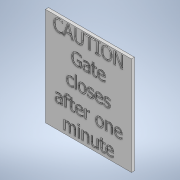
# Autodesk Inventor part: warningSignV2
Saved by Autodesk Inventor 2021.2 (Build 252289000, 289)
## iProperties
Created: 2020-11-24
Part Number: warningSignV2
Material: Generic
Document SubType Name: Modeling
Designer: robst
Density: 1 g/cm^3
Appearance: Default
Author: robst
Autodesk Inventor part; units mm, degrees
ref_plane "YZ Plane" through (0, 0, 0) normal (1, 0, 0) x (0, 1, 0)
ref_plane "XZ Plane" through (0, 0, 0) normal (0, 1, 0) x (-1, 0, 0)
ref_plane "XY Plane" through (0, 0, 0) normal (0, 0, 1) x (1, 0, 0)
sketch "Sketch4" plane through (0, 0, 0) normal (0, 0, 1) x (1, 0, 0)
  line L0 (-88.9, -101.6) -> (88.9, -101.6)
  line L1 (88.9, -101.6) -> (88.9, 101.6)
  line L2 (88.9, 101.6) -> (-88.9, 101.6)
  line L3 (-88.9, 101.6) -> (-88.9, -101.6)
  line L4 (-88.9, -101.6) -> (88.9, 101.6) construction
  line L5 (88.9, -101.6) -> (-88.9, 101.6) construction
  point P0 (0, 0)
  dimension "d12" = 203.2
  dimension "d13" = 177.8
  constraints: 12 end point, 2 midpoint, 2 parallel, 1 horizontal, 1 perpendicular
  measures "d12" distance of L2.end L0.start
  measures "d13" distance of L0.start L0.end
extrude "Extrusion2" add sketch "Sketch4" against normal blind 6.35
sketch "Sketch5" plane through (0, 0, 0) normal (0, 0, 1) x (1, 0, 0)
  line L0 (-88.9, -101.6) -> (-88.9, 101.6) construction
  line L1 (-88.9, 73.66) -> (88.9, 73.66) construction
  line L2 (88.9, 101.6) -> (88.9, -101.6) construction
  line L3 (88.9, 101.6) -> (-88.9, 101.6) construction
  spline S0 degree 2 poles (-60.6595, 73.2072) (-63.1295, 73.2072) (-67.3079, 74.8744) (-68.8311, 76.5417) knots 0 0 0 1 2 2 2
  spline S1 degree 2 poles (-68.8311, 76.5417) (-70.3543, 78.1884) (-72.0216, 83.1284) (-72.0216, 86.3394) knots 0 0 0 1 2 2 2
  spline S2 degree 2 poles (-72.0216, 86.3394) (-72.0216, 89.5299) (-70.3955, 94.2641) (-68.8517, 96.0136) knots 0 0 0 1 2 2 2
  spline S3 degree 2 poles (-68.8517, 96.0136) (-67.3285, 97.7221) (-63.1707, 99.5128) (-60.5977, 99.5128) knots 0 0 0 1 2 2 2
  spline S4 degree 2 poles (-60.5977, 99.5128) (-59.3216, 99.5128) (-57.078, 99.1423) (-56.1311, 98.8542) knots 0 0 0 1 2 2 2
  spline S5 degree 2 poles (-56.1311, 98.8542) (-55.3078, 98.5866) (-53.5993, 97.825) (-52.7554, 97.3722) knots 0 0 0 1 2 2 2
  line L4 (-52.7554, 97.3722) -> (-52.7554, 93.2966)
  line L5 (-52.7554, 93.2966) -> (-53.023, 93.2966)
  spline S6 degree 2 poles (-53.023, 93.2966) (-53.4758, 93.7083) (-54.8755, 94.861) (-55.8841, 95.4167) knots 0 0 0 1 2 2 2
  spline S7 degree 2 poles (-55.8841, 95.4167) (-56.8515, 95.9519) (-59.1363, 96.6312) (-60.6183, 96.6312) knots 0 0 0 1 2 2 2
  spline S8 degree 2 poles (-60.6183, 96.6312) (-62.2444, 96.6312) (-65.1467, 95.2932) (-66.2376, 94.017) knots 0 0 0 1 2 2 2
  spline S9 degree 2 poles (-66.2376, 94.017) (-67.3079, 92.7203) (-68.5018, 88.7888) (-68.5018, 86.3394) knots 0 0 0 1 2 2 2
  spline S10 degree 2 poles (-68.5018, 86.3394) (-68.5018, 83.7253) (-67.2462, 79.9585) (-66.1553, 78.6618) knots 0 0 0 1 2 2 2
  spline S11 degree 2 poles (-66.1553, 78.6618) (-65.0849, 77.4062) (-62.2238, 76.13) (-60.6183, 76.13) knots 0 0 0 1 2 2 2
  spline S12 degree 2 poles (-60.6183, 76.13) (-59.1569, 76.13) (-56.6663, 76.8504) (-55.6989, 77.3856) knots 0 0 0 1 2 2 2
  spline S13 degree 2 poles (-55.6989, 77.3856) (-54.7726, 77.9208) (-53.3935, 79.0323) (-53.0024, 79.4234) knots 0 0 0 1 2 2 2
  line L6 (-53.0024, 79.4234) -> (-52.7554, 79.4234)
  line L7 (-52.7554, 79.4234) -> (-52.7554, 75.389)
  spline S14 degree 2 poles (-52.7554, 75.389) (-53.5993, 74.9979) (-55.0814, 74.2775) (-56.1311, 73.9482) knots 0 0 0 1 2 2 2
  spline S15 degree 2 poles (-56.1311, 73.9482) (-57.2426, 73.5777) (-59.1363, 73.2072) (-60.6595, 73.2072) knots 0 0 0 1 2 2 2
  line L8 (-52.3438, 73.66) -> (-43.781, 99.06)
  line L9 (-43.781, 99.06) -> (-39.6232, 99.06)
  line L10 (-39.6232, 99.06) -> (-31.0605, 73.66)
  line L11 (-31.0605, 73.66) -> (-34.6214, 73.66)
  line L12 (-34.6214, 73.66) -> (-36.9267, 80.7613)
  line L13 (-36.9267, 80.7613) -> (-46.6216, 80.7613)
  line L14 (-46.6216, 80.7613) -> (-48.9269, 73.66)
  line L15 (-48.9269, 73.66) -> (-52.3438, 73.66)
  line L16 (-37.853, 83.643) -> (-41.7844, 95.602)
  line L17 (-41.7844, 95.602) -> (-45.6953, 83.643)
  line L18 (-45.6953, 83.643) -> (-37.853, 83.643)
  spline S16 degree 2 poles (-19.4514, 73.1248) (-21.695, 73.1248) (-25.0295, 74.2981) (-26.2028, 75.4713) knots 0 0 0 1 2 2 2
  spline S17 degree 2 poles (-26.2028, 75.4713) (-27.5407, 76.7887) (-28.6316, 80.4937) (-28.6316, 83.2107) knots 0 0 0 1 2 2 2
  line L19 (-28.6316, 83.2107) -> (-28.6316, 99.06)
  line L20 (-28.6316, 99.06) -> (-25.2559, 99.06)
  line L21 (-25.2559, 99.06) -> (-25.2559, 83.2107)
  spline S18 degree 2 poles (-25.2559, 83.2107) (-25.2559, 81.4406) (-24.8031, 79.0529) (-24.165, 78.0854) knots 0 0 0 1 2 2 2
  spline S19 degree 2 poles (-24.165, 78.0854) (-23.4857, 77.0563) (-21.1392, 76.0065) (-19.4514, 76.0065) knots 0 0 0 1 2 2 2
  spline S20 degree 2 poles (-19.4514, 76.0065) (-17.8665, 76.0065) (-15.3964, 77.0563) (-14.7172, 78.0854) knots 0 0 0 1 2 2 2
  spline S21 degree 2 poles (-14.7172, 78.0854) (-14.0791, 79.0529) (-13.6263, 81.42) (-13.6263, 83.1284) knots 0 0 0 1 2 2 2
  line L22 (-13.6263, 83.1284) -> (-13.6263, 99.06)
  line L23 (-13.6263, 99.06) -> (-10.2506, 99.06)
  line L24 (-10.2506, 99.06) -> (-10.2506, 83.2107)
  spline S22 degree 2 poles (-10.2506, 83.2107) (-10.2506, 80.5555) (-11.3209, 76.7681) (-12.6794, 75.4713) knots 0 0 0 1 2 2 2
  spline S23 degree 2 poles (-12.6794, 75.4713) (-13.8938, 74.2775) (-17.1049, 73.1248) (-19.4514, 73.1248) knots 0 0 0 1 2 2 2
  line L25 (0.5146, 73.66) -> (0.5146, 96.0548)
  line L26 (0.5146, 96.0548) -> (-8.007, 96.0548)
  line L27 (-8.007, 96.0548) -> (-8.007, 99.06)
  line L28 (-8.007, 99.06) -> (12.4118, 99.06)
  line L29 (12.4118, 99.06) -> (12.4118, 96.0548)
  line L30 (12.4118, 96.0548) -> (3.8903, 96.0548)
  line L31 (3.8903, 96.0548) -> (3.8903, 73.66)
  line L32 (3.8903, 73.66) -> (0.5146, 73.66)
  line L33 (23.8562, 73.66) -> (14.0173, 73.66)
  line L34 (14.0173, 73.66) -> (14.0173, 76.2535)
  line L35 (14.0173, 76.2535) -> (17.2489, 76.2535)
  line L36 (17.2489, 76.2535) -> (17.2489, 96.4665)
  line L37 (17.2489, 96.4665) -> (14.0173, 96.4665)
  line L38 (14.0173, 96.4665) -> (14.0173, 99.06)
  line L39 (14.0173, 99.06) -> (23.8562, 99.06)
  line L40 (23.8562, 99.06) -> (23.8562, 96.4665)
  line L41 (23.8562, 96.4665) -> (20.6246, 96.4665)
  line L42 (20.6246, 96.4665) -> (20.6246, 76.2535)
  line L43 (20.6246, 76.2535) -> (23.8562, 76.2535)
  line L44 (23.8562, 76.2535) -> (23.8562, 73.66)
  spline S24 degree 2 poles (46.004, 96.1577) (47.4449, 94.4699) (49.0504, 89.5299) (49.0504, 86.36) knots 0 0 0 1 2 2 2
  spline S25 degree 2 poles (49.0504, 86.36) (49.0504, 83.2725) (47.4861, 78.2707) (46.004, 76.5829) knots 0 0 0 1 2 2 2
  spline S26 degree 2 poles (46.004, 76.5829) (44.4397, 74.8127) (40.3024, 73.1248) (37.8118, 73.1248) knots 0 0 0 1 2 2 2
  spline S27 degree 2 poles (37.8118, 73.1248) (35.2389, 73.1248) (31.1222, 74.8744) (29.6196, 76.5829) knots 0 0 0 1 2 2 2
  spline S28 degree 2 poles (29.6196, 76.5829) (28.1582, 78.2707) (26.5938, 83.2313) (26.5938, 86.36) knots 0 0 0 1 2 2 2
  spline S29 degree 2 poles (26.5938, 86.36) (26.5938, 89.5504) (28.1788, 94.4081) (29.6402, 96.1577) knots 0 0 0 1 2 2 2
  spline S30 degree 2 poles (29.6402, 96.1577) (31.1222, 97.8456) (35.2595, 99.5952) (37.8118, 99.5952) knots 0 0 0 1 2 2 2
  spline S31 degree 2 poles (37.8118, 99.5952) (40.4053, 99.5952) (44.5632, 97.7838) (46.004, 96.1577) knots 0 0 0 1 2 2 2
  spline S32 degree 2 poles (45.5306, 86.36) (45.5306, 88.8712) (44.4397, 92.7615) (43.4517, 94.0376) knots 0 0 0 1 2 2 2
  spline S33 degree 2 poles (43.4517, 94.0376) (42.4431, 95.355) (39.6026, 96.6723) (37.8324, 96.6723) knots 0 0 0 1 2 2 2
  spline S34 degree 2 poles (37.8324, 96.6723) (36.0005, 96.6723) (33.2423, 95.3961) (32.1925, 94.0376) knots 0 0 0 1 2 2 2
  spline S35 degree 2 poles (32.1925, 94.0376) (31.184, 92.7409) (30.1136, 88.83) (30.1136, 86.36) knots 0 0 0 1 2 2 2
  spline S36 degree 2 poles (30.1136, 86.36) (30.1136, 81.3582) (34.3126, 76.0477) (37.8324, 76.0477) knots 0 0 0 1 2 2 2
  spline S37 degree 2 poles (37.8324, 76.0477) (41.3522, 76.0477) (45.5306, 81.3582) (45.5306, 86.36) knots 0 0 0 1 2 2 2
  line L45 (70.9306, 73.66) -> (67.1433, 73.66)
  line L46 (67.1433, 73.66) -> (55.9047, 95.5608)
  line L47 (55.9047, 95.5608) -> (55.9047, 73.66)
  line L48 (55.9047, 73.66) -> (52.7554, 73.66)
  line L49 (52.7554, 73.66) -> (52.7554, 99.06)
  line L50 (52.7554, 99.06) -> (57.5514, 99.06)
  line L51 (57.5514, 99.06) -> (67.7814, 78.95)
  line L52 (67.7814, 78.95) -> (67.7814, 99.06)
  line L53 (67.7814, 99.06) -> (70.9306, 99.06)
  line L54 (70.9306, 99.06) -> (70.9306, 73.66)
  spline S38 degree 2 poles (-22.6521, 31.3038) (-25.3485, 31.3038) (-29.8152, 32.9505) (-31.4207, 34.6177) knots 0 0 0 1 2 2 2
  spline S39 degree 2 poles (-31.4207, 34.6177) (-33.0262, 36.3056) (-34.7346, 41.2868) (-34.7346, 44.5184) knots 0 0 0 1 2 2 2
  spline S40 degree 2 poles (-34.7346, 44.5184) (-34.7346, 47.5853) (-33.0056, 52.443) (-31.4001, 54.172) knots 0 0 0 1 2 2 2
  spline S41 degree 2 poles (-31.4001, 54.172) (-29.8563, 55.8393) (-25.328, 57.6506) (-22.6315, 57.6506) knots 0 0 0 1 2 2 2
  spline S42 degree 2 poles (-22.6315, 57.6506) (-21.3348, 57.6506) (-18.9882, 57.2801) (-17.9179, 56.9508) knots 0 0 0 1 2 2 2
  spline S43 degree 2 poles (-17.9179, 56.9508) (-17.0534, 56.7038) (-14.9539, 55.7981) (-14.3158, 55.4688) knots 0 0 0 1 2 2 2
  line L55 (-14.3158, 55.4688) -> (-14.3158, 51.3933)
  line L56 (-14.3158, 51.3933) -> (-14.604, 51.3933)
  spline S44 degree 2 poles (-14.604, 51.3933) (-15.2421, 51.949) (-16.58, 52.9576) (-17.815, 53.534) knots 0 0 0 1 2 2 2
  spline S45 degree 2 poles (-17.815, 53.534) (-18.8442, 54.0485) (-21.4994, 54.7278) (-23.0226, 54.7278) knots 0 0 0 1 2 2 2
  spline S46 degree 2 poles (-23.0226, 54.7278) (-26.6865, 54.7278) (-31.2148, 49.2114) (-31.2148, 44.6213) knots 0 0 0 1 2 2 2
  spline S47 degree 2 poles (-31.2148, 44.6213) (-31.2148, 42.069) (-30.021, 38.2404) (-28.8889, 36.9231) knots 0 0 0 1 2 2 2
  spline S48 degree 2 poles (-28.8889, 36.9231) (-27.798, 35.6058) (-24.7105, 34.2267) (-22.7756, 34.2267) knots 0 0 0 1 2 2 2
  spline S49 degree 2 poles (-22.7756, 34.2267) (-21.3553, 34.2267) (-18.5148, 34.6383) (-17.5474, 35.05) knots 0 0 0 1 2 2 2
  line L57 (-17.5474, 35.05) -> (-17.5474, 41.6161)
  line L58 (-17.5474, 41.6161) -> (-23.4343, 41.6161)
  line L59 (-23.4343, 41.6161) -> (-23.4343, 44.5801)
  line L60 (-23.4343, 44.5801) -> (-14.2129, 44.5801)
  line L61 (-14.2129, 44.5801) -> (-14.2129, 33.4857)
  spline S50 degree 2 poles (-14.2129, 33.4857) (-14.851, 33.1975) (-17.0328, 32.3124) (-17.9591, 32.0448) knots 0 0 0 1 2 2 2
  spline S51 degree 2 poles (-17.9591, 32.0448) (-19.2147, 31.6743) (-21.2318, 31.3038) (-22.6521, 31.3038) knots 0 0 0 1 2 2 2
  spline S52 degree 2 poles (0.4014, 33.815) (0.0103, 33.5268) (-1.3071, 32.4976) (-1.9246, 32.1889) knots 0 0 0 1 2 2 2
  spline S53 degree 2 poles (-1.9246, 32.1889) (-2.7685, 31.7361) (-4.3534, 31.2626) (-5.7942, 31.2626) knots 0 0 0 1 2 2 2
  spline S54 degree 2 poles (-5.7942, 31.2626) (-6.9675, 31.2626) (-9.0876, 32.1477) (-9.8904, 32.9505) knots 0 0 0 1 2 2 2
  spline S55 degree 2 poles (-9.8904, 32.9505) (-10.6519, 33.7327) (-11.5782, 36.038) (-11.5782, 37.3142) knots 0 0 0 1 2 2 2
  spline S56 degree 2 poles (-11.5782, 37.3142) (-11.5782, 39.2902) (-9.9109, 42.0895) (-8.0996, 42.8923) knots 0 0 0 1 2 2 2
  spline S57 degree 2 poles (-8.0996, 42.8923) (-6.4941, 43.6333) (-2.1304, 44.1891) (0.4014, 44.3331) knots 0 0 0 1 2 2 2
  line L62 (0.4014, 44.3331) -> (0.4014, 44.9506)
  spline S58 degree 2 poles (0.4014, 44.9506) (0.4014, 46.0622) (-0.2779, 47.4412) (-0.8954, 47.8323) knots 0 0 0 1 2 2 2
  spline S59 degree 2 poles (-0.8954, 47.8323) (-1.5129, 48.2234) (-3.2831, 48.4704) (-4.2299, 48.4704) knots 0 0 0 1 2 2 2
  spline S60 degree 2 poles (-4.2299, 48.4704) (-5.3414, 48.4704) (-8.3466, 47.8117) (-9.8492, 47.1737) knots 0 0 0 1 2 2 2
  line L63 (-9.8492, 47.1737) -> (-10.0344, 47.1737)
  line L64 (-10.0344, 47.1737) -> (-10.0344, 50.4464)
  spline S61 degree 2 poles (-10.0344, 50.4464) (-9.1494, 50.6934) (-5.8354, 51.3109) (-4.2093, 51.3109) knots 0 0 0 1 2 2 2
  spline S62 degree 2 poles (-4.2093, 51.3109) (-2.2333, 51.3109) (0.4631, 50.6934) (1.5335, 49.8907) knots 0 0 0 1 2 2 2
  spline S63 degree 2 poles (1.5335, 49.8907) (2.5832, 49.1085) (3.6124, 46.6179) (3.6124, 44.8271) knots 0 0 0 1 2 2 2
  line L65 (3.6124, 44.8271) -> (3.6124, 31.7978)
  line L66 (3.6124, 31.7978) -> (0.4014, 31.7978)
  line L67 (0.4014, 31.7978) -> (0.4014, 33.815)
  line L68 (0.4014, 36.4908) -> (0.4014, 41.7808)
  spline S64 degree 2 poles (0.4014, 41.7808) (-0.7513, 41.6779) (-4.2299, 41.328) (-5.3208, 40.9986) knots 0 0 0 1 2 2 2
  spline S65 degree 2 poles (-5.3208, 40.9986) (-6.597, 40.6075) (-8.2643, 38.9814) (-8.2643, 37.5406) knots 0 0 0 1 2 2 2
  spline S66 degree 2 poles (-8.2643, 37.5406) (-8.2643, 35.8939) (-6.4118, 34.2267) (-4.6416, 34.2267) knots 0 0 0 1 2 2 2
  spline S67 degree 2 poles (-4.6416, 34.2267) (-3.139, 34.2267) (-0.669, 35.5234) (0.4014, 36.4908) knots 0 0 0 1 2 2 2
  spline S68 degree 2 poles (13.8835, 31.4273) (11.2694, 31.4273) (8.326, 34.4119) (8.326, 37.6435) knots 0 0 0 1 2 2 2
  line L69 (8.326, 37.6435) -> (8.326, 48.2028)
  line L70 (8.326, 48.2028) -> (6.1647, 48.2028)
  line L71 (6.1647, 48.2028) -> (6.1647, 50.8581)
  line L72 (6.1647, 50.8581) -> (8.326, 50.8581)
  line L73 (8.326, 50.8581) -> (8.326, 56.3333)
  line L74 (8.326, 56.3333) -> (11.537, 56.3333)
  line L75 (11.537, 56.3333) -> (11.537, 50.8581)
  line L76 (11.537, 50.8581) -> (17.4445, 50.8581)
  line L77 (17.4445, 50.8581) -> (17.4445, 48.2028)
  line L78 (17.4445, 48.2028) -> (11.537, 48.2028)
  line L79 (11.537, 48.2028) -> (11.537, 39.1255)
  spline S69 degree 2 poles (11.537, 39.1255) (11.537, 37.6847) (11.64, 36.0998) (11.9899, 35.4205) knots 0 0 0 1 2 2 2
  spline S70 degree 2 poles (11.9899, 35.4205) (12.278, 34.8236) (13.5748, 34.2267) (14.6863, 34.2267) knots 0 0 0 1 2 2 2
  spline S71 degree 2 poles (14.6863, 34.2267) (15.4685, 34.2267) (16.9299, 34.7001) (17.2592, 34.8442) knots 0 0 0 1 2 2 2
  line L80 (17.2592, 34.8442) -> (17.4445, 34.8442)
  line L81 (17.4445, 34.8442) -> (17.4445, 31.9625)
  spline S72 degree 2 poles (17.4445, 31.9625) (16.5388, 31.7155) (14.6863, 31.4273) (13.8835, 31.4273) knots 0 0 0 1 2 2 2
  spline S73 degree 2 poles (28.0861, 31.3656) (23.5166, 31.3656) (18.4942, 36.4908) (18.4942, 41.225) knots 0 0 0 1 2 2 2
  spline S74 degree 2 poles (18.4942, 41.225) (18.4942, 45.8769) (23.3725, 51.3933) (27.304, 51.3933) knots 0 0 0 1 2 2 2
  spline S75 degree 2 poles (27.304, 51.3933) (29.0741, 51.3933) (31.8117, 50.3641) (32.8203, 49.2732) knots 0 0 0 1 2 2 2
  spline S76 degree 2 poles (32.8203, 49.2732) (33.8495, 48.1823) (34.9404, 45.033) (34.9404, 42.7482) knots 0 0 0 1 2 2 2
  line L82 (34.9404, 42.7482) -> (34.9404, 40.9986)
  line L83 (34.9404, 40.9986) -> (21.7464, 40.9986)
  spline S77 degree 2 poles (21.7464, 40.9986) (21.7464, 37.6847) (25.081, 34.1649) (28.045, 34.1649) knots 0 0 0 1 2 2 2
  spline S78 degree 2 poles (28.045, 34.1649) (29.0947, 34.1649) (31.1325, 34.6383) (31.9558, 35.0088) knots 0 0 0 1 2 2 2
  spline S79 degree 2 poles (31.9558, 35.0088) (32.8203, 35.4205) (34.0142, 36.1409) (34.4053, 36.4703) knots 0 0 0 1 2 2 2
  line L84 (34.4053, 36.4703) -> (34.5905, 36.4703)
  line L85 (34.5905, 36.4703) -> (34.5905, 32.9711)
  spline S80 degree 2 poles (34.5905, 32.9711) (34.0348, 32.7446) (32.3469, 32.086) (31.6882, 31.9007) knots 0 0 0 1 2 2 2
  spline S81 degree 2 poles (31.6882, 31.9007) (30.762, 31.6331) (29.2388, 31.3656) (28.0861, 31.3656) knots 0 0 0 1 2 2 2
  spline S82 degree 2 poles (31.8117, 43.4481) (31.7706, 44.7448) (31.2354, 46.6385) (30.7208, 47.2766) knots 0 0 0 1 2 2 2
  spline S83 degree 2 poles (30.7208, 47.2766) (30.1651, 47.997) (28.4155, 48.7586) (27.1187, 48.7586) knots 0 0 0 1 2 2 2
  spline S84 degree 2 poles (27.1187, 48.7586) (25.8425, 48.7586) (24.0518, 47.997) (23.3108, 47.256) knots 0 0 0 1 2 2 2
  spline S85 degree 2 poles (23.3108, 47.256) (22.5904, 46.4944) (21.8494, 44.6625) (21.7464, 43.4481) knots 0 0 0 1 2 2 2
  line L86 (21.7464, 43.4481) -> (31.8117, 43.4481)
  spline S86 degree 2 poles (-36.4019, -11.1759) (-38.3779, -11.1759) (-41.6506, -9.9615) (-42.8239, -8.7265) knots 0 0 0 1 2 2 2
  spline S87 degree 2 poles (-42.8239, -8.7265) (-43.9972, -7.512) (-45.2939, -3.7658) (-45.2939, -1.2547) knots 0 0 0 1 2 2 2
  spline S88 degree 2 poles (-45.2939, -1.2547) (-45.2939, 1.2565) (-43.956, 4.9204) (-42.8239, 6.1554) knots 0 0 0 1 2 2 2
  spline S89 degree 2 poles (-42.8239, 6.1554) (-41.6918, 7.411) (-38.3367, 8.7489) (-36.4019, 8.7489) knots 0 0 0 1 2 2 2
  spline S90 degree 2 poles (-36.4019, 8.7489) (-34.8375, 8.7489) (-31.9147, 7.8638) (-30.7826, 7.2875) knots 0 0 0 1 2 2 2
  line L87 (-30.7826, 7.2875) -> (-30.7826, 3.6854)
  line L88 (-30.7826, 3.6854) -> (-30.9678, 3.6854)
  spline S91 degree 2 poles (-30.9678, 3.6854) (-31.3177, 3.9735) (-32.3881, 4.7146) (-33.1497, 5.1056) knots 0 0 0 1 2 2 2
  spline S92 degree 2 poles (-33.1497, 5.1056) (-33.8289, 5.435) (-35.6403, 5.9496) (-36.4636, 5.9496) knots 0 0 0 1 2 2 2
  spline S93 degree 2 poles (-36.4636, 5.9496) (-38.9542, 5.9496) (-41.98, 2.1828) (-41.98, -1.2547) knots 0 0 0 1 2 2 2
  spline S94 degree 2 poles (-41.98, -1.2547) (-41.98, -4.6098) (-39.0571, -8.3765) (-36.4636, -8.3765) knots 0 0 0 1 2 2 2
  spline S95 degree 2 poles (-36.4636, -8.3765) (-34.8993, -8.3765) (-32.0587, -7.0798) (-30.9678, -6.0712) knots 0 0 0 1 2 2 2
  line L89 (-30.9678, -6.0712) -> (-30.7826, -6.0712)
  line L90 (-30.7826, -6.0712) -> (-30.7826, -9.6733)
  spline S96 degree 2 poles (-30.7826, -9.6733) (-31.256, -9.8997) (-32.6968, -10.5378) (-33.2732, -10.6819) knots 0 0 0 1 2 2 2
  spline S97 degree 2 poles (-33.2732, -10.6819) (-34.0965, -10.9289) (-35.3933, -11.1759) (-36.4019, -11.1759) knots 0 0 0 1 2 2 2
  line L91 (-24.587, -10.7436) -> (-27.798, -10.7436)
  line L92 (-27.798, -10.7436) -> (-27.798, 15.7885)
  line L93 (-27.798, 15.7885) -> (-24.587, 15.7885)
  line L94 (-24.587, 15.7885) -> (-24.587, -10.7436)
  spline S98 degree 2 poles (-4.2093, -1.2135) (-4.2093, -6.03) (-8.8406, -11.2788) (-12.7103, -11.2788) knots 0 0 0 1 2 2 2
  spline S99 degree 2 poles (-12.7103, -11.2788) (-16.6829, -11.2788) (-21.2318, -5.8654) (-21.2318, -1.2135) knots 0 0 0 1 2 2 2
  spline S100 degree 2 poles (-21.2318, -1.2135) (-21.2318, 3.5619) (-16.5388, 8.8518) (-12.7103, 8.8518) knots 0 0 0 1 2 2 2
  spline S101 degree 2 poles (-12.7103, 8.8518) (-8.8406, 8.8518) (-4.2093, 3.5825) (-4.2093, -1.2135) knots 0 0 0 1 2 2 2
  spline S102 degree 2 poles (-7.5233, -1.2135) (-7.5233, 2.4915) (-10.2197, 6.0936) (-12.7103, 6.0936) knots 0 0 0 1 2 2 2
  spline S103 degree 2 poles (-12.7103, 6.0936) (-15.2009, 6.0936) (-17.9179, 2.4915) (-17.9179, -1.2135) knots 0 0 0 1 2 2 2
  spline S104 degree 2 poles (-17.9179, -1.2135) (-17.9179, -4.8156) (-15.2009, -8.5206) (-12.7103, -8.5206) knots 0 0 0 1 2 2 2
  spline S105 degree 2 poles (-12.7103, -8.5206) (-10.2403, -8.5206) (-7.5233, -4.8773) (-7.5233, -1.2135) knots 0 0 0 1 2 2 2
  spline S106 degree 2 poles (4.2299, -11.1965) (2.3156, -11.1965) (-0.9983, -10.1673) (-2.0892, -9.591) knots 0 0 0 1 2 2 2
  line L95 (-2.0892, -9.591) -> (-2.0892, -5.9889)
  line L96 (-2.0892, -5.9889) -> (-1.9246, -5.9889)
  spline S107 degree 2 poles (-1.9246, -5.9889) (-1.5129, -6.3182) (-0.4014, -7.1004) (0.5249, -7.5326) knots 0 0 0 1 2 2 2
  spline S108 degree 2 poles (0.5249, -7.5326) (1.3276, -7.9237) (3.3036, -8.5) (4.3534, -8.5) knots 0 0 0 1 2 2 2
  spline S109 degree 2 poles (4.3534, -8.5) (5.115, -8.5) (6.8646, -8.1501) (7.2763, -7.8619) knots 0 0 0 1 2 2 2
  spline S110 degree 2 poles (7.2763, -7.8619) (7.8732, -7.4709) (8.4083, -6.5858) (8.4083, -5.6801) knots 0 0 0 1 2 2 2
  spline S111 degree 2 poles (8.4083, -5.6801) (8.4083, -4.548) (7.1733, -3.3748) (5.5884, -2.9837) knots 0 0 0 1 2 2 2
  spline S112 degree 2 poles (5.5884, -2.9837) (4.9709, -2.8396) (2.9949, -2.4279) (2.151, -2.2015) knots 0 0 0 1 2 2 2
  spline S113 degree 2 poles (2.151, -2.2015) (-0.0309, -1.5634) (-2.0069, 1.0713) (-2.0069, 2.9444) knots 0 0 0 1 2 2 2
  spline S114 degree 2 poles (-2.0069, 2.9444) (-2.0069, 5.5379) (1.8834, 8.7695) (5.0944, 8.7695) knots 0 0 0 1 2 2 2
  spline S115 degree 2 poles (5.0944, 8.7695) (6.6793, 8.7695) (9.8904, 7.9873) (10.9813, 7.3904) knots 0 0 0 1 2 2 2
  line L97 (10.9813, 7.3904) -> (10.9813, 3.953)
  line L98 (10.9813, 3.953) -> (10.8166, 3.953)
  spline S116 degree 2 poles (10.8166, 3.953) (9.5816, 4.941) (6.5764, 6.0731) (5.0327, 6.0731) knots 0 0 0 1 2 2 2
  spline S117 degree 2 poles (5.0327, 6.0731) (3.4477, 6.0731) (1.2659, 4.7351) (1.2659, 3.3972) knots 0 0 0 1 2 2 2
  spline S118 degree 2 poles (1.2659, 3.3972) (1.2659, 2.1828) (2.5626, 1.0095) (4.0035, 0.639) knots 0 0 0 1 2 2 2
  spline S119 degree 2 poles (4.0035, 0.639) (4.7033, 0.4538) (6.4735, 0.0833) (7.4409, -0.1431) knots 0 0 0 1 2 2 2
  spline S120 degree 2 poles (7.4409, -0.1431) (9.5404, -0.6783) (11.6811, -3.1278) (11.6811, -5.2478) knots 0 0 0 1 2 2 2
  spline S121 degree 2 poles (11.6811, -5.2478) (11.6811, -6.4829) (10.7137, -8.6647) (9.7669, -9.4675) knots 0 0 0 1 2 2 2
  spline S122 degree 2 poles (9.7669, -9.4675) (8.7583, -10.3114) (6.1853, -11.1965) (4.2299, -11.1965) knots 0 0 0 1 2 2 2
  spline S123 degree 2 poles (22.9403, -11.1759) (18.3707, -11.1759) (13.3484, -6.0506) (13.3484, -1.3164) knots 0 0 0 1 2 2 2
  spline S124 degree 2 poles (13.3484, -1.3164) (13.3484, 3.3355) (18.2267, 8.8518) (22.1581, 8.8518) knots 0 0 0 1 2 2 2
  spline S125 degree 2 poles (22.1581, 8.8518) (23.9283, 8.8518) (26.6659, 7.8227) (27.6745, 6.7317) knots 0 0 0 1 2 2 2
  spline S126 degree 2 poles (27.6745, 6.7317) (28.7036, 5.6408) (29.7946, 2.4915) (29.7946, 0.2068) knots 0 0 0 1 2 2 2
  line L99 (29.7946, 0.2068) -> (29.7946, -1.5428)
  line L100 (29.7946, -1.5428) -> (16.6006, -1.5428)
  spline S127 degree 2 poles (16.6006, -1.5428) (16.6006, -4.8568) (19.9351, -8.3765) (22.8991, -8.3765) knots 0 0 0 1 2 2 2
  spline S128 degree 2 poles (22.8991, -8.3765) (23.9489, -8.3765) (25.9866, -7.9031) (26.81, -7.5326) knots 0 0 0 1 2 2 2
  spline S129 degree 2 poles (26.81, -7.5326) (27.6745, -7.1209) (28.8683, -6.4005) (29.2594, -6.0712) knots 0 0 0 1 2 2 2
  line L101 (29.2594, -6.0712) -> (29.4447, -6.0712)
  line L102 (29.4447, -6.0712) -> (29.4447, -9.5704)
  spline S130 degree 2 poles (29.4447, -9.5704) (28.8889, -9.7968) (27.2011, -10.4555) (26.5424, -10.6407) knots 0 0 0 1 2 2 2
  spline S131 degree 2 poles (26.5424, -10.6407) (25.6161, -10.9083) (24.093, -11.1759) (22.9403, -11.1759) knots 0 0 0 1 2 2 2
  spline S132 degree 2 poles (26.6659, 0.9066) (26.6247, 2.2034) (26.0895, 4.097) (25.575, 4.7351) knots 0 0 0 1 2 2 2
  spline S133 degree 2 poles (25.575, 4.7351) (25.0192, 5.4556) (23.2696, 6.2171) (21.9729, 6.2171) knots 0 0 0 1 2 2 2
  spline S134 degree 2 poles (21.9729, 6.2171) (20.6967, 6.2171) (18.9059, 5.4556) (18.1649, 4.7146) knots 0 0 0 1 2 2 2
  spline S135 degree 2 poles (18.1649, 4.7146) (17.4445, 3.953) (16.7035, 2.121) (16.6006, 0.9066) knots 0 0 0 1 2 2 2
  line L103 (16.6006, 0.9066) -> (26.6659, 0.9066)
  spline S136 degree 2 poles (38.1926, -11.1965) (36.2784, -11.1965) (32.9644, -10.1673) (31.8735, -9.591) knots 0 0 0 1 2 2 2
  line L104 (31.8735, -9.591) -> (31.8735, -5.9889)
  line L105 (31.8735, -5.9889) -> (32.0382, -5.9889)
  spline S137 degree 2 poles (32.0382, -5.9889) (32.4498, -6.3182) (33.5613, -7.1004) (34.4876, -7.5326) knots 0 0 0 1 2 2 2
  spline S138 degree 2 poles (34.4876, -7.5326) (35.2904, -7.9237) (37.2664, -8.5) (38.3161, -8.5) knots 0 0 0 1 2 2 2
  spline S139 degree 2 poles (38.3161, -8.5) (39.0777, -8.5) (40.8273, -8.1501) (41.239, -7.8619) knots 0 0 0 1 2 2 2
  spline S140 degree 2 poles (41.239, -7.8619) (41.8359, -7.4709) (42.3711, -6.5858) (42.3711, -5.6801) knots 0 0 0 1 2 2 2
  spline S141 degree 2 poles (42.3711, -5.6801) (42.3711, -4.548) (41.1361, -3.3748) (39.5511, -2.9837) knots 0 0 0 1 2 2 2
  spline S142 degree 2 poles (39.5511, -2.9837) (38.9336, -2.8396) (36.9576, -2.4279) (36.1137, -2.2015) knots 0 0 0 1 2 2 2
  spline S143 degree 2 poles (36.1137, -2.2015) (33.9318, -1.5634) (31.9558, 1.0713) (31.9558, 2.9444) knots 0 0 0 1 2 2 2
  spline S144 degree 2 poles (31.9558, 2.9444) (31.9558, 5.5379) (35.8461, 8.7695) (39.0571, 8.7695) knots 0 0 0 1 2 2 2
  spline S145 degree 2 poles (39.0571, 8.7695) (40.6421, 8.7695) (43.8531, 7.9873) (44.944, 7.3904) knots 0 0 0 1 2 2 2
  line L106 (44.944, 7.3904) -> (44.944, 3.953)
  line L107 (44.944, 3.953) -> (44.7793, 3.953)
  spline S146 degree 2 poles (44.7793, 3.953) (43.5443, 4.941) (40.5391, 6.0731) (38.9954, 6.0731) knots 0 0 0 1 2 2 2
  spline S147 degree 2 poles (38.9954, 6.0731) (37.4105, 6.0731) (35.2286, 4.7351) (35.2286, 3.3972) knots 0 0 0 1 2 2 2
  spline S148 degree 2 poles (35.2286, 3.3972) (35.2286, 2.1828) (36.5254, 1.0095) (37.9662, 0.639) knots 0 0 0 1 2 2 2
  spline S149 degree 2 poles (37.9662, 0.639) (38.666, 0.4538) (40.4362, 0.0833) (41.4036, -0.1431) knots 0 0 0 1 2 2 2
  spline S150 degree 2 poles (41.4036, -0.1431) (43.5032, -0.6783) (45.6438, -3.1278) (45.6438, -5.2478) knots 0 0 0 1 2 2 2
  spline S151 degree 2 poles (45.6438, -5.2478) (45.6438, -6.4829) (44.6764, -8.6647) (43.7296, -9.4675) knots 0 0 0 1 2 2 2
  spline S152 degree 2 poles (43.7296, -9.4675) (42.721, -10.3114) (40.1481, -11.1965) (38.1926, -11.1965) knots 0 0 0 1 2 2 2
  spline S153 degree 2 poles (-56.975, -51.4326) (-57.3661, -51.7207) (-58.6835, -52.7499) (-59.301, -53.0587) knots 0 0 0 1 2 2 2
  spline S154 degree 2 poles (-59.301, -53.0587) (-60.1449, -53.5115) (-61.7298, -53.9849) (-63.1707, -53.9849) knots 0 0 0 1 2 2 2
  spline S155 degree 2 poles (-63.1707, -53.9849) (-64.3439, -53.9849) (-66.464, -53.0998) (-67.2668, -52.2971) knots 0 0 0 1 2 2 2
  spline S156 degree 2 poles (-67.2668, -52.2971) (-68.0284, -51.5149) (-68.9546, -49.2096) (-68.9546, -47.9334) knots 0 0 0 1 2 2 2
  spline S157 degree 2 poles (-68.9546, -47.9334) (-68.9546, -45.9574) (-67.2874, -43.158) (-65.476, -42.3553) knots 0 0 0 1 2 2 2
  spline S158 degree 2 poles (-65.476, -42.3553) (-63.8705, -41.6143) (-59.5068, -41.0585) (-56.975, -40.9144) knots 0 0 0 1 2 2 2
  line L108 (-56.975, -40.9144) -> (-56.975, -40.2969)
  spline S159 degree 2 poles (-56.975, -40.2969) (-56.975, -39.1854) (-57.6543, -37.8063) (-58.2718, -37.4152) knots 0 0 0 1 2 2 2
  spline S160 degree 2 poles (-58.2718, -37.4152) (-58.8893, -37.0241) (-60.6595, -36.7771) (-61.6063, -36.7771) knots 0 0 0 1 2 2 2
  spline S161 degree 2 poles (-61.6063, -36.7771) (-62.7178, -36.7771) (-65.723, -37.4358) (-67.2256, -38.0739) knots 0 0 0 1 2 2 2
  line L109 (-67.2256, -38.0739) -> (-67.4109, -38.0739)
  line L110 (-67.4109, -38.0739) -> (-67.4109, -34.8011)
  spline S162 degree 2 poles (-67.4109, -34.8011) (-66.5258, -34.5541) (-63.2118, -33.9366) (-61.5857, -33.9366) knots 0 0 0 1 2 2 2
  spline S163 degree 2 poles (-61.5857, -33.9366) (-59.6097, -33.9366) (-56.9133, -34.5541) (-55.8429, -35.3569) knots 0 0 0 1 2 2 2
  spline S164 degree 2 poles (-55.8429, -35.3569) (-54.7932, -36.1391) (-53.764, -38.6296) (-53.764, -40.4204) knots 0 0 0 1 2 2 2
  line L111 (-53.764, -40.4204) -> (-53.764, -53.4497)
  line L112 (-53.764, -53.4497) -> (-56.975, -53.4497)
  line L113 (-56.975, -53.4497) -> (-56.975, -51.4326)
  line L114 (-56.975, -48.7567) -> (-56.975, -43.4668)
  spline S165 degree 2 poles (-56.975, -43.4668) (-58.1277, -43.5697) (-61.6063, -43.9196) (-62.6972, -44.2489) knots 0 0 0 1 2 2 2
  spline S166 degree 2 poles (-62.6972, -44.2489) (-63.9734, -44.64) (-65.6407, -46.2661) (-65.6407, -47.707) knots 0 0 0 1 2 2 2
  spline S167 degree 2 poles (-65.6407, -47.707) (-65.6407, -49.3536) (-63.7882, -51.0209) (-62.018, -51.0209) knots 0 0 0 1 2 2 2
  spline S168 degree 2 poles (-62.018, -51.0209) (-60.5154, -51.0209) (-58.0454, -49.7241) (-56.975, -48.7567) knots 0 0 0 1 2 2 2
  line L115 (-39.2321, -30.0052) -> (-39.3968, -30.0052)
  spline S169 degree 2 poles (-39.3968, -30.0052) (-39.829, -29.8405) (-41.4345, -29.5523) (-42.0726, -29.5523) knots 0 0 0 1 2 2 2
  spline S170 degree 2 poles (-42.0726, -29.5523) (-44.0898, -29.5523) (-45.8188, -31.3637) (-45.8188, -33.7514) knots 0 0 0 1 2 2 2
  line L116 (-45.8188, -33.7514) -> (-45.8188, -34.3895)
  line L117 (-45.8188, -34.3895) -> (-40.5083, -34.3895)
  line L118 (-40.5083, -34.3895) -> (-40.5083, -37.0447)
  line L119 (-40.5083, -37.0447) -> (-45.7159, -37.0447)
  line L120 (-45.7159, -37.0447) -> (-45.7159, -53.4497)
  line L121 (-45.7159, -53.4497) -> (-48.9269, -53.4497)
  line L122 (-48.9269, -53.4497) -> (-48.9269, -37.0447)
  line L123 (-48.9269, -37.0447) -> (-51.0882, -37.0447)
  line L124 (-51.0882, -37.0447) -> (-51.0882, -34.3895)
  line L125 (-51.0882, -34.3895) -> (-48.9269, -34.3895)
  line L126 (-48.9269, -34.3895) -> (-48.9269, -33.7514)
  spline S171 degree 2 poles (-48.9269, -33.7514) (-48.9269, -30.3345) (-45.613, -26.753) (-42.5254, -26.753) knots 0 0 0 1 2 2 2
  spline S172 degree 2 poles (-42.5254, -26.753) (-41.6404, -26.753) (-39.9319, -26.9382) (-39.2321, -27.0617) knots 0 0 0 1 2 2 2
  line L127 (-39.2321, -27.0617) -> (-39.2321, -30.0052)
  spline S173 degree 2 poles (-31.6368, -53.8202) (-34.2509, -53.8202) (-37.1943, -50.8356) (-37.1943, -47.604) knots 0 0 0 1 2 2 2
  line L128 (-37.1943, -47.604) -> (-37.1943, -37.0447)
  line L129 (-37.1943, -37.0447) -> (-39.3556, -37.0447)
  line L130 (-39.3556, -37.0447) -> (-39.3556, -34.3895)
  line L131 (-39.3556, -34.3895) -> (-37.1943, -34.3895)
  line L132 (-37.1943, -34.3895) -> (-37.1943, -28.9143)
  line L133 (-37.1943, -28.9143) -> (-33.9833, -28.9143)
  line L134 (-33.9833, -28.9143) -> (-33.9833, -34.3895)
  line L135 (-33.9833, -34.3895) -> (-28.0758, -34.3895)
  line L136 (-28.0758, -34.3895) -> (-28.0758, -37.0447)
  line L137 (-28.0758, -37.0447) -> (-33.9833, -37.0447)
  line L138 (-33.9833, -37.0447) -> (-33.9833, -46.122)
  spline S174 degree 2 poles (-33.9833, -46.122) (-33.9833, -47.5629) (-33.8804, -49.1478) (-33.5305, -49.8271) knots 0 0 0 1 2 2 2
  spline S175 degree 2 poles (-33.5305, -49.8271) (-33.2423, -50.424) (-31.9455, -51.0209) (-30.834, -51.0209) knots 0 0 0 1 2 2 2
  spline S176 degree 2 poles (-30.834, -51.0209) (-30.0519, -51.0209) (-28.5904, -50.5475) (-28.2611, -50.4034) knots 0 0 0 1 2 2 2
  line L139 (-28.2611, -50.4034) -> (-28.0758, -50.4034)
  line L140 (-28.0758, -50.4034) -> (-28.0758, -53.2851)
  spline S177 degree 2 poles (-28.0758, -53.2851) (-28.9815, -53.5321) (-30.834, -53.8202) (-31.6368, -53.8202) knots 0 0 0 1 2 2 2
  spline S178 degree 2 poles (-17.4342, -53.882) (-22.0037, -53.882) (-27.0261, -48.7567) (-27.0261, -44.0225) knots 0 0 0 1 2 2 2
  spline S179 degree 2 poles (-27.0261, -44.0225) (-27.0261, -39.3707) (-22.1478, -33.8543) (-18.2164, -33.8543) knots 0 0 0 1 2 2 2
  spline S180 degree 2 poles (-18.2164, -33.8543) (-16.4462, -33.8543) (-13.7086, -34.8835) (-12.7, -35.9744) knots 0 0 0 1 2 2 2
  spline S181 degree 2 poles (-12.7, -35.9744) (-11.6708, -37.0653) (-10.5799, -40.2146) (-10.5799, -42.4993) knots 0 0 0 1 2 2 2
  line L141 (-10.5799, -42.4993) -> (-10.5799, -44.2489)
  line L142 (-10.5799, -44.2489) -> (-23.7739, -44.2489)
  spline S182 degree 2 poles (-23.7739, -44.2489) (-23.7739, -47.5629) (-20.4394, -51.0826) (-17.4754, -51.0826) knots 0 0 0 1 2 2 2
  spline S183 degree 2 poles (-17.4754, -51.0826) (-16.4256, -51.0826) (-14.3878, -50.6092) (-13.5645, -50.2387) knots 0 0 0 1 2 2 2
  spline S184 degree 2 poles (-13.5645, -50.2387) (-12.7, -49.8271) (-11.5062, -49.1066) (-11.1151, -48.7773) knots 0 0 0 1 2 2 2
  line L143 (-11.1151, -48.7773) -> (-10.9298, -48.7773)
  line L144 (-10.9298, -48.7773) -> (-10.9298, -52.2765)
  spline S185 degree 2 poles (-10.9298, -52.2765) (-11.4856, -52.5029) (-13.1734, -53.1616) (-13.8321, -53.3468) knots 0 0 0 1 2 2 2
  spline S186 degree 2 poles (-13.8321, -53.3468) (-14.7583, -53.6144) (-16.2815, -53.882) (-17.4342, -53.882) knots 0 0 0 1 2 2 2
  spline S187 degree 2 poles (-13.7086, -41.7995) (-13.7498, -40.5027) (-14.2849, -38.6091) (-14.7995, -37.971) knots 0 0 0 1 2 2 2
  spline S188 degree 2 poles (-14.7995, -37.971) (-15.3553, -37.2506) (-17.1049, -36.489) (-18.4016, -36.489) knots 0 0 0 1 2 2 2
  spline S189 degree 2 poles (-18.4016, -36.489) (-19.6778, -36.489) (-21.4686, -37.2506) (-22.2096, -37.9916) knots 0 0 0 1 2 2 2
  spline S190 degree 2 poles (-22.2096, -37.9916) (-22.93, -38.7532) (-23.671, -40.5851) (-23.7739, -41.7995) knots 0 0 0 1 2 2 2
  line L145 (-23.7739, -41.7995) -> (-13.7086, -41.7995)
  line L146 (2.7788, -37.8269) -> (2.6141, -37.8269)
  spline S191 degree 2 poles (2.6141, -37.8269) (2.2436, -37.724) (1.4408, -37.6828) (0.8851, -37.6828) knots 0 0 0 1 2 2 2
  spline S192 degree 2 poles (0.8851, -37.6828) (-0.4117, -37.6828) (-2.964, -38.8149) (-4.1167, -39.9264) knots 0 0 0 1 2 2 2
  line L147 (-4.1167, -39.9264) -> (-4.1167, -53.4497)
  line L148 (-4.1167, -53.4497) -> (-7.3277, -53.4497)
  line L149 (-7.3277, -53.4497) -> (-7.3277, -34.3895)
  line L150 (-7.3277, -34.3895) -> (-4.1167, -34.3895)
  line L151 (-4.1167, -34.3895) -> (-4.1167, -37.23)
  spline S193 degree 2 poles (-4.1167, -37.23) (-2.3671, -35.6656) (0.247, -34.3895) (1.482, -34.3895) knots 0 0 0 1 2 2 2
  spline S194 degree 2 poles (1.482, -34.3895) (1.976, -34.3895) (2.47, -34.4306) (2.7788, -34.4924) knots 0 0 0 1 2 2 2
  line L152 (2.7788, -34.4924) -> (2.7788, -37.8269)
  spline S195 degree 2 poles (31.8426, -43.9196) (31.8426, -48.7361) (27.2113, -53.9849) (23.3417, -53.9849) knots 0 0 0 1 2 2 2
  spline S196 degree 2 poles (23.3417, -53.9849) (19.369, -53.9849) (14.8201, -48.5715) (14.8201, -43.9196) knots 0 0 0 1 2 2 2
  spline S197 degree 2 poles (14.8201, -43.9196) (14.8201, -39.1442) (19.5131, -33.8543) (23.3417, -33.8543) knots 0 0 0 1 2 2 2
  spline S198 degree 2 poles (23.3417, -33.8543) (27.2113, -33.8543) (31.8426, -39.1237) (31.8426, -43.9196) knots 0 0 0 1 2 2 2
  spline S199 degree 2 poles (28.5287, -43.9196) (28.5287, -40.2146) (25.8323, -36.6125) (23.3417, -36.6125) knots 0 0 0 1 2 2 2
  spline S200 degree 2 poles (23.3417, -36.6125) (20.8511, -36.6125) (18.134, -40.2146) (18.134, -43.9196) knots 0 0 0 1 2 2 2
  spline S201 degree 2 poles (18.134, -43.9196) (18.134, -47.5217) (20.8511, -51.2267) (23.3417, -51.2267) knots 0 0 0 1 2 2 2
  spline S202 degree 2 poles (23.3417, -51.2267) (25.8117, -51.2267) (28.5287, -47.5835) (28.5287, -43.9196) knots 0 0 0 1 2 2 2
  line L153 (50.1002, -53.4497) -> (46.8891, -53.4497)
  line L154 (46.8891, -53.4497) -> (46.8891, -42.5817)
  spline S203 degree 2 poles (46.8891, -42.5817) (46.8891, -41.2643) (46.6421, -39.0002) (46.2716, -38.3209) knots 0 0 0 1 2 2 2
  spline S204 degree 2 poles (46.2716, -38.3209) (45.8806, -37.6005) (44.4809, -36.9006) (43.287, -36.9006) knots 0 0 0 1 2 2 2
  spline S205 degree 2 poles (43.287, -36.9006) (42.0932, -36.9006) (39.5614, -38.1768) (38.347, -39.206) knots 0 0 0 1 2 2 2
  line L155 (38.347, -39.206) -> (38.347, -53.4497)
  line L156 (38.347, -53.4497) -> (35.136, -53.4497)
  line L157 (35.136, -53.4497) -> (35.136, -34.3895)
  line L158 (35.136, -34.3895) -> (38.347, -34.3895)
  line L159 (38.347, -34.3895) -> (38.347, -36.5096)
  spline S206 degree 2 poles (38.347, -36.5096) (39.7878, -35.2128) (42.5666, -33.8543) (44.131, -33.8543) knots 0 0 0 1 2 2 2
  spline S207 degree 2 poles (44.131, -33.8543) (46.9303, -33.8543) (50.1002, -37.5593) (50.1002, -41.0791) knots 0 0 0 1 2 2 2
  line L160 (50.1002, -41.0791) -> (50.1002, -53.4497)
  spline S208 degree 2 poles (62.8825, -53.882) (58.313, -53.882) (53.2906, -48.7567) (53.2906, -44.0225) knots 0 0 0 1 2 2 2
  spline S209 degree 2 poles (53.2906, -44.0225) (53.2906, -39.3707) (58.1689, -33.8543) (62.1003, -33.8543) knots 0 0 0 1 2 2 2
  spline S210 degree 2 poles (62.1003, -33.8543) (63.8705, -33.8543) (66.6081, -34.8835) (67.6167, -35.9744) knots 0 0 0 1 2 2 2
  spline S211 degree 2 poles (67.6167, -35.9744) (68.6459, -37.0653) (69.7368, -40.2146) (69.7368, -42.4993) knots 0 0 0 1 2 2 2
  line L161 (69.7368, -42.4993) -> (69.7368, -44.2489)
  line L162 (69.7368, -44.2489) -> (56.5428, -44.2489)
  spline S212 degree 2 poles (56.5428, -44.2489) (56.5428, -47.5629) (59.8773, -51.0826) (62.8413, -51.0826) knots 0 0 0 1 2 2 2
  spline S213 degree 2 poles (62.8413, -51.0826) (63.8911, -51.0826) (65.9288, -50.6092) (66.7522, -50.2387) knots 0 0 0 1 2 2 2
  spline S214 degree 2 poles (66.7522, -50.2387) (67.6167, -49.8271) (68.8105, -49.1066) (69.2016, -48.7773) knots 0 0 0 1 2 2 2
  line L163 (69.2016, -48.7773) -> (69.3869, -48.7773)
  line L164 (69.3869, -48.7773) -> (69.3869, -52.2765)
  spline S215 degree 2 poles (69.3869, -52.2765) (68.8311, -52.5029) (67.1433, -53.1616) (66.4846, -53.3468) knots 0 0 0 1 2 2 2
  spline S216 degree 2 poles (66.4846, -53.3468) (65.5583, -53.6144) (64.0352, -53.882) (62.8825, -53.882) knots 0 0 0 1 2 2 2
  spline S217 degree 2 poles (66.6081, -41.7995) (66.5669, -40.5027) (66.0318, -38.6091) (65.5172, -37.971) knots 0 0 0 1 2 2 2
  spline S218 degree 2 poles (65.5172, -37.971) (64.9614, -37.2506) (63.2118, -36.489) (61.9151, -36.489) knots 0 0 0 1 2 2 2
  spline S219 degree 2 poles (61.9151, -36.489) (60.6389, -36.489) (58.8481, -37.2506) (58.1071, -37.9916) knots 0 0 0 1 2 2 2
  spline S220 degree 2 poles (58.1071, -37.9916) (57.3867, -38.7532) (56.6457, -40.5851) (56.5428, -41.7995) knots 0 0 0 1 2 2 2
  line L165 (56.5428, -41.7995) -> (66.6081, -41.7995)
  line L166 (-29.2285, -95.0238) -> (-29.2285, -83.991)
  spline S221 degree 2 poles (-29.2285, -83.991) (-29.2285, -82.6737) (-29.4344, -80.4301) (-29.7637, -79.8126) knots 0 0 0 1 2 2 2
  spline S222 degree 2 poles (-29.7637, -79.8126) (-30.093, -79.1333) (-31.3486, -78.4747) (-32.4395, -78.4747) knots 0 0 0 1 2 2 2
  spline S223 degree 2 poles (-32.4395, -78.4747) (-33.4275, -78.4747) (-35.6917, -79.6891) (-36.8856, -80.8418) knots 0 0 0 1 2 2 2
  spline S224 degree 2 poles (-36.8856, -80.8418) (-36.865, -81.1299) (-36.8238, -81.9327) (-36.8238, -82.4679) knots 0 0 0 1 2 2 2
  line L167 (-36.8238, -82.4679) -> (-36.8238, -95.0238)
  line L168 (-36.8238, -95.0238) -> (-40.0348, -95.0238)
  line L169 (-40.0348, -95.0238) -> (-40.0348, -83.991)
  spline S225 degree 2 poles (-40.0348, -83.991) (-40.0348, -82.6737) (-40.2407, -80.4301) (-40.57, -79.8126) knots 0 0 0 1 2 2 2
  spline S226 degree 2 poles (-40.57, -79.8126) (-40.8993, -79.1333) (-42.1549, -78.4747) (-43.2459, -78.4747) knots 0 0 0 1 2 2 2
  spline S227 degree 2 poles (-43.2459, -78.4747) (-44.275, -78.4747) (-46.5598, -79.7714) (-47.6301, -80.78) knots 0 0 0 1 2 2 2
  line L170 (-47.6301, -80.78) -> (-47.6301, -95.0238)
  line L171 (-47.6301, -95.0238) -> (-50.8412, -95.0238)
  line L172 (-50.8412, -95.0238) -> (-50.8412, -75.9635)
  line L173 (-50.8412, -75.9635) -> (-47.6301, -75.9635)
  line L174 (-47.6301, -75.9635) -> (-47.6301, -78.063)
  spline S228 degree 2 poles (-47.6301, -78.063) (-46.3746, -76.8074) (-43.9045, -75.4283) (-42.4225, -75.4283) knots 0 0 0 1 2 2 2
  spline S229 degree 2 poles (-42.4225, -75.4283) (-40.7347, -75.4283) (-38.1206, -76.9721) (-37.4413, -78.7217) knots 0 0 0 1 2 2 2
  spline S230 degree 2 poles (-37.4413, -78.7217) (-35.9799, -77.0956) (-33.2217, -75.4283) (-31.6162, -75.4283) knots 0 0 0 1 2 2 2
  spline S231 degree 2 poles (-31.6162, -75.4283) (-30.3812, -75.4283) (-28.364, -76.1899) (-27.623, -77.0544) knots 0 0 0 1 2 2 2
  spline S232 degree 2 poles (-27.623, -77.0544) (-26.8614, -77.9189) (-26.0175, -80.5124) (-26.0175, -82.4679) knots 0 0 0 1 2 2 2
  line L175 (-26.0175, -82.4679) -> (-26.0175, -95.0238)
  line L176 (-26.0175, -95.0238) -> (-29.2285, -95.0238)
  line L177 (-18.237, -95.0238) -> (-21.448, -95.0238)
  line L178 (-21.448, -95.0238) -> (-21.448, -75.9635)
  line L179 (-21.448, -75.9635) -> (-18.237, -75.9635)
  line L180 (-18.237, -75.9635) -> (-18.237, -95.0238)
  line L181 (-18.0105, -72.7936) -> (-21.6538, -72.7936)
  line L182 (-21.6538, -72.7936) -> (-21.6538, -69.4591)
  line L183 (-21.6538, -69.4591) -> (-18.0105, -69.4591)
  line L184 (-18.0105, -69.4591) -> (-18.0105, -72.7936)
  line L185 (1.4408, -95.0238) -> (-1.7702, -95.0238)
  line L186 (-1.7702, -95.0238) -> (-1.7702, -84.1557)
  spline S233 degree 2 poles (-1.7702, -84.1557) (-1.7702, -82.8384) (-2.0172, -80.5742) (-2.3877, -79.8949) knots 0 0 0 1 2 2 2
  spline S234 degree 2 poles (-2.3877, -79.8949) (-2.7788, -79.1745) (-4.1784, -78.4747) (-5.3723, -78.4747) knots 0 0 0 1 2 2 2
  spline S235 degree 2 poles (-5.3723, -78.4747) (-6.5661, -78.4747) (-9.0979, -79.7508) (-10.3123, -80.78) knots 0 0 0 1 2 2 2
  line L187 (-10.3123, -80.78) -> (-10.3123, -95.0238)
  line L188 (-10.3123, -95.0238) -> (-13.5233, -95.0238)
  line L189 (-13.5233, -95.0238) -> (-13.5233, -75.9635)
  line L190 (-13.5233, -75.9635) -> (-10.3123, -75.9635)
  line L191 (-10.3123, -75.9635) -> (-10.3123, -78.0836)
  spline S236 degree 2 poles (-10.3123, -78.0836) (-8.8715, -76.7868) (-6.0927, -75.4283) (-4.5284, -75.4283) knots 0 0 0 1 2 2 2
  spline S237 degree 2 poles (-4.5284, -75.4283) (-1.729, -75.4283) (1.4408, -79.1333) (1.4408, -82.6531) knots 0 0 0 1 2 2 2
  line L192 (1.4408, -82.6531) -> (1.4408, -95.0238)
  line L193 (20.7687, -95.0238) -> (17.5577, -95.0238)
  line L194 (17.5577, -95.0238) -> (17.5577, -92.9243)
  spline S238 degree 2 poles (17.5577, -92.9243) (16.0757, -94.221) (13.4204, -95.5589) (11.7737, -95.5589) knots 0 0 0 1 2 2 2
  spline S239 degree 2 poles (11.7737, -95.5589) (10.5387, -95.5589) (8.3363, -94.7356) (7.5335, -93.8505) knots 0 0 0 1 2 2 2
  spline S240 degree 2 poles (7.5335, -93.8505) (6.7102, -92.9654) (5.8045, -90.269) (5.8045, -88.3341) knots 0 0 0 1 2 2 2
  line L195 (5.8045, -88.3341) -> (5.8045, -75.9635)
  line L196 (5.8045, -75.9635) -> (9.0156, -75.9635)
  line L197 (9.0156, -75.9635) -> (9.0156, -86.8315)
  spline S241 degree 2 poles (9.0156, -86.8315) (9.0156, -88.3547) (9.242, -90.3513) (9.6331, -91.0923) knots 0 0 0 1 2 2 2
  spline S242 degree 2 poles (9.6331, -91.0923) (10.0241, -91.8333) (11.3621, -92.5126) (12.6177, -92.5126) knots 0 0 0 1 2 2 2
  spline S243 degree 2 poles (12.6177, -92.5126) (13.7909, -92.5126) (16.4462, -91.1747) (17.5577, -90.2072) knots 0 0 0 1 2 2 2
  line L198 (17.5577, -90.2072) -> (17.5577, -75.9635)
  line L199 (17.5577, -75.9635) -> (20.7687, -75.9635)
  line L200 (20.7687, -75.9635) -> (20.7687, -95.0238)
  spline S244 degree 2 poles (31.184, -95.3943) (28.5699, -95.3943) (25.6264, -92.4097) (25.6264, -89.1781) knots 0 0 0 1 2 2 2
  line L201 (25.6264, -89.1781) -> (25.6264, -78.6187)
  line L202 (25.6264, -78.6187) -> (23.4652, -78.6187)
  line L203 (23.4652, -78.6187) -> (23.4652, -75.9635)
  line L204 (23.4652, -75.9635) -> (25.6264, -75.9635)
  line L205 (25.6264, -75.9635) -> (25.6264, -70.4883)
  line L206 (25.6264, -70.4883) -> (28.8374, -70.4883)
  line L207 (28.8374, -70.4883) -> (28.8374, -75.9635)
  line L208 (28.8374, -75.9635) -> (34.7449, -75.9635)
  line L209 (34.7449, -75.9635) -> (34.7449, -78.6187)
  line L210 (34.7449, -78.6187) -> (28.8374, -78.6187)
  line L211 (28.8374, -78.6187) -> (28.8374, -87.6961)
  spline S245 degree 2 poles (28.8374, -87.6961) (28.8374, -89.1369) (28.9404, -90.7218) (29.2903, -91.4011) knots 0 0 0 1 2 2 2
  spline S246 degree 2 poles (29.2903, -91.4011) (29.5784, -91.998) (30.8752, -92.5949) (31.9867, -92.5949) knots 0 0 0 1 2 2 2
  spline S247 degree 2 poles (31.9867, -92.5949) (32.7689, -92.5949) (34.2303, -92.1215) (34.5596, -91.9774) knots 0 0 0 1 2 2 2
  line L212 (34.5596, -91.9774) -> (34.7449, -91.9774)
  line L213 (34.7449, -91.9774) -> (34.7449, -94.8591)
  spline S248 degree 2 poles (34.7449, -94.8591) (33.8392, -95.1061) (31.9867, -95.3943) (31.184, -95.3943) knots 0 0 0 1 2 2 2
  spline S249 degree 2 poles (45.3865, -95.456) (40.817, -95.456) (35.7947, -90.3307) (35.7947, -85.5965) knots 0 0 0 1 2 2 2
  spline S250 degree 2 poles (35.7947, -85.5965) (35.7947, -80.9447) (40.6729, -75.4283) (44.6044, -75.4283) knots 0 0 0 1 2 2 2
  spline S251 degree 2 poles (44.6044, -75.4283) (46.3746, -75.4283) (49.1122, -76.4575) (50.1207, -77.5484) knots 0 0 0 1 2 2 2
  spline S252 degree 2 poles (50.1207, -77.5484) (51.1499, -78.6393) (52.2408, -81.7886) (52.2408, -84.0734) knots 0 0 0 1 2 2 2
  line L214 (52.2408, -84.0734) -> (52.2408, -85.823)
  line L215 (52.2408, -85.823) -> (39.0468, -85.823)
  spline S253 degree 2 poles (39.0468, -85.823) (39.0468, -89.1369) (42.3814, -92.6567) (45.3454, -92.6567) knots 0 0 0 1 2 2 2
  spline S254 degree 2 poles (45.3454, -92.6567) (46.3951, -92.6567) (48.4329, -92.1832) (49.2562, -91.8127) knots 0 0 0 1 2 2 2
  spline S255 degree 2 poles (49.2562, -91.8127) (50.1207, -91.4011) (51.3146, -90.6807) (51.7057, -90.3513) knots 0 0 0 1 2 2 2
  line L216 (51.7057, -90.3513) -> (51.8909, -90.3513)
  line L217 (51.8909, -90.3513) -> (51.8909, -93.8505)
  spline S256 degree 2 poles (51.8909, -93.8505) (51.3352, -94.0769) (49.6473, -94.7356) (48.9887, -94.9208) knots 0 0 0 1 2 2 2
  spline S257 degree 2 poles (48.9887, -94.9208) (48.0624, -95.1884) (46.5392, -95.456) (45.3865, -95.456) knots 0 0 0 1 2 2 2
  spline S258 degree 2 poles (49.1122, -83.3735) (49.071, -82.0768) (48.5358, -80.1831) (48.0212, -79.545) knots 0 0 0 1 2 2 2
  spline S259 degree 2 poles (48.0212, -79.545) (47.4655, -78.8246) (45.7159, -78.063) (44.4191, -78.063) knots 0 0 0 1 2 2 2
  spline S260 degree 2 poles (44.4191, -78.063) (43.1429, -78.063) (41.3522, -78.8246) (40.6112, -79.5656) knots 0 0 0 1 2 2 2
  spline S261 degree 2 poles (40.6112, -79.5656) (39.8908, -80.3272) (39.1498, -82.1591) (39.0468, -83.3735) knots 0 0 0 1 2 2 2
  line L218 (39.0468, -83.3735) -> (49.1122, -83.3735)
  point P0 (0, 0)
  dimension "d16" = 27.94
  constraints: 2 end point, 2 horizontal, 2 point on line
  measures "d16" distance between parallel lines of L1 L3
emboss "Emboss2" sketch "Sketch5" operation cut depth 2.54 direction (0, 0, -1)
body "Solid2"
